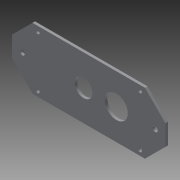
# Autodesk Inventor part: ToughBox Nano AM14U2 Mount
Saved by Autodesk Inventor 2015 SP1 (Build 190203100, 203)
## iProperties
Created: 2015-01-10
Part Number: ToughBox Nano AM14U2 Mount
Material: Generic
Document SubType Name: Modeling
Designer: Jarod
Density: 1 g/cm^3
Appearance: Default
Author: Jarod
Autodesk Inventor part; units mm, degrees
ref_plane "YZ Plane" through (0, 0, 0) normal (1, 0, 0) x (0, 1, 0)
ref_plane "XZ Plane" through (0, 0, 0) normal (0, 1, 0) x (-1, 0, 0)
ref_plane "XY Plane" through (0, 0, 0) normal (0, 0, 1) x (1, 0, 0)
sketch "Sketch1" plane through (0, 0, 0) normal (0, 0, 1) x (1, 0, 0)
  line L0 (0, 0) -> (139.7, 0)
  line L1 (139.7, 0) -> (139.7, 76.2)
  line L2 (139.7, 76.2) -> (0, 76.2)
  line L3 (0, 76.2) -> (0, 0)
  dimension "d0" = 139.7
  dimension "d1" = 76.2
  constraints: 8 end point, 2 parallel, 1 horizontal, 1 perpendicular
  measures "d0" distance of L2.end L1.end
  measures "d1" distance of L1.end L0.end
extrude "Extrusion1" add sketch "Sketch1" along normal blind 3.175
sketch "Sketch2" plane through (0, 0, 3.175) normal (0, 0, 1) x (1, 0, 0)
  line L0 (0, 0) -> (139.7, 0) projected
  line L1 (139.7, 0) -> (139.7, 76.2) projected
  line L2 (139.7, 76.2) -> (0, 76.2) projected
  line L3 (0, 76.2) -> (0, 0) projected
  circle A0 centre (6.35, 69.85) radius 2.54
  circle A1 centre (6.35, 6.35) radius 2.54
  circle A2 centre (133.35, 6.35) radius 2.54
  circle A3 centre (133.35, 69.85) radius 2.54
  circle A4 centre (63.5, 38.1) radius 11.1125
  circle A5 centre (104.14, 38.1) radius 14.2875
  dimension "d4" = 6.35
  dimension "d5" = 6.35
  dimension "d6" = 69.85
  dimension "d7" = 6.35
  dimension "d8" = 133.35
  dimension "d9" = 6.35
  dimension "d10" = 133.35
  dimension "d11" = 69.85
  dimension "d12" = 63.5
  dimension "d13" = 38.1
  dimension "d14" = 38.1
  dimension "d15" = 104.14
  dimension "d16" = 5.08
  dimension "d17" = 5.08
  dimension "d18" = 5.08
  dimension "d19" = 5.08
  dimension "d20" = 22.225
  dimension "d21" = 28.575
  constraints: 6 centre point, 6 coincident
  measures "d4" horizontal distance of point (0, 0) point (6.35, 6.35)
  measures "d5" horizontal distance of point (6.35, 6.35) point (0, 0)
  measures "d6" vertical distance of point (6.35, 69.85) point (0, 0)
  measures "d7" horizontal distance of point (6.35, 69.85) point (0, 0)
  measures "d8" horizontal distance of point (133.35, 6.35) point (0, 0)
  measures "d9" vertical distance of point (133.35, 6.35) point (0, 0)
  measures "d10" horizontal distance of point (133.35, 69.85) point (0, 0)
  measures "d11" vertical distance of point (133.35, 69.85) point (0, 0)
  measures "d12" horizontal distance of point (0, 0) point (63.5, 38.1)
  measures "d13" vertical distance of point (0, 0) point (63.5, 38.1)
  measures "d14" vertical distance of point (0, 0) point (104.14, 38.1)
  measures "d15" horizontal distance of point (0, 0) point (104.14, 38.1)
  measures "d16" diameter of A0
  measures "d17" diameter of A1
  measures "d18" diameter of A2
  measures "d19" diameter of A3
  measures "d20" diameter of A4
  measures "d21" diameter of A5
extrude "Extrusion2" cut sketch "Sketch2" against normal blind 3.175 contours A0 | A1 | A2 | A3 | A4 | A5
sketch "Sketch3" plane through (0, 0, 3.175) normal (0, 0, 1) x (1, 0, 0)
  circle A0 centre (63.5, 38.1) radius 11.1125 projected
  circle A1 centre (133.35, 6.35) radius 2.54 projected
  circle A2 centre (6.35, 69.85) radius 2.54 projected
  circle A3 centre (6.35, 6.35) radius 2.54 projected
  circle A4 centre (133.35, 69.85) radius 2.54 projected
  circle A5 centre (104.14, 38.1) radius 14.2875 projected
  line L0 (0, 0) -> (139.7, 0) projected
  line L1 (139.7, 0) -> (139.7, 76.2) projected
  line L2 (139.7, 76.2) -> (0, 76.2) projected
  line L3 (0, 76.2) -> (0, 0) projected
  line L4 (0, 76.2) -> (0, 0) projected
  line L5 (0, 25.4) -> (-25.4, 25.4)
  line L6 (-25.4, 25.4) -> (-25.4, 50.8)
  line L7 (-25.4, 50.8) -> (0, 50.8)
  line L8 (0, 50.8) -> (0, 25.4)
  line L9 (0, 76.2) -> (-25.4, 50.8)
  line L10 (-25.4, 25.4) -> (0, 0)
  line L11 (139.7, 0) -> (139.7, 76.2) projected
  line L12 (139.7, 50.8) -> (165.1, 50.8)
  line L13 (165.1, 50.8) -> (165.1, 25.4)
  line L14 (165.1, 25.4) -> (139.7, 25.4)
  line L15 (139.7, 25.4) -> (139.7, 50.8)
  line L16 (0, 76.2) -> (0, 50.8)
  line L17 (0, 0) -> (0, 25.4)
  line L18 (139.7, 76.2) -> (139.7, 50.8)
  line L19 (165.1, 50.8) -> (139.7, 76.2)
  line L20 (165.1, 25.4) -> (139.7, 0)
  line L21 (139.7, 0) -> (139.7, 25.4)
  dimension "d24" = 25.4
  dimension "d25" = 25.4
  dimension "d26" = 25.4
  dimension "d27" = 25.4
  dimension "d28" = 25.4
  dimension "d29" = 25.4
  constraints: 32 end point, 5 parallel, 3 perpendicular, 2 collinear, 2 horizontal, 2 point on line
  measures "d24" distance between parallel lines of L7 L5
  measures "d25" distance between parallel lines of L3 L6
  measures "d26" distance from line of L5 L4.end
  measures "d27" distance of L13.end L14.end
  measures "d28" distance from line of L4.end L14
  measures "d29" distance between parallel lines of L14 L12
extrude "Extrusion3" add sketch "Sketch3" against normal blind 3.175 contours L10 L5 L3 | L1 L14 L20 | L5 L6 L7 L3 | L1 L12 L13 L14 | L7 L9 L3 | L1 L19 L12
sketch "Sketch4" plane through (0, 0, 3.175) normal (0, 0, 1) x (1, 0, 0)
  circle A0 centre (63.5, 38.1) radius 11.1125 projected
  circle A1 centre (133.35, 6.35) radius 2.54 projected
  circle A2 centre (6.35, 69.85) radius 2.54 projected
  circle A3 centre (6.35, 6.35) radius 2.54 projected
  circle A4 centre (133.35, 69.85) radius 2.54 projected
  circle A5 centre (104.14, 38.1) radius 14.2875 projected
  line L0 (0, 0) -> (139.7, 0) projected
  line L1 (139.7, 0) -> (165.1, 25.4) projected
  line L2 (165.1, 25.4) -> (165.1, 50.8) projected
  line L3 (165.1, 50.8) -> (139.7, 76.2) projected
  line L4 (139.7, 76.2) -> (0, 76.2) projected
  line L5 (0, 76.2) -> (-25.4, 50.8) projected
  line L6 (-25.4, 50.8) -> (-25.4, 25.4) projected
  line L7 (-25.4, 25.4) -> (0, 0) projected
  circle A6 centre (-12.7, 38.1) radius 3.175
  circle A7 centre (152.4, 38.1) radius 3.175
  dimension "d32" = 6.35
  dimension "d33" = 12.7
  dimension "d34" = 38.1
  dimension "d35" = 6.35
  dimension "d36" = 152.4
  dimension "d37" = 38.1
  constraints: 2 centre point
  measures "d32" diameter of A6
  measures "d33" horizontal distance of A6.centre point (0, 0)
  measures "d34" vertical distance of point (0, 0) A6.centre
  measures "d35" diameter of A7
  measures "d36" horizontal distance of A7.centre point (0, 0)
  measures "d37" vertical distance of point (0, 0) A7.centre
extrude "Extrusion4" cut sketch "Sketch4" against normal blind 3.175 contours A6 | A7
body "Solid1"
